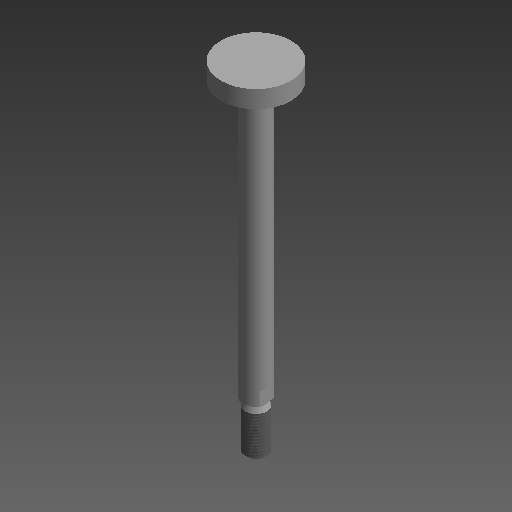
# Autodesk Inventor part: 193992 DSNU-32-60-PPS---(A---00--0-KS)
Saved by Autodesk Inventor 2021 (Build 250183000, 183)
## iProperties
Part Number: 193992 DSNU-32-60-PPS---(A---00--0-KS)
Material: Generic
Catalog Web Link: www.cadenas.de
Description: DSNU---(KS)-Standard cylinder
Vendor: FESTO
Document SubType Name: Modeling
Designer: partserver
Manufacturer: FESTO
Mass: 22.1775 g
Surface Area: 78.0411 cm^2
Volume: 22.1775 cm^3
Density: 1 g/cm^3
Appearance: PSOLRGB-192-192-192
Category: PARTsolutions
Company: FESTO
PSOL_IDENT_0: {$CADENAS_DATA\23d-libs\festo\parts\d\dsnu\parts\dsnu_metric_ks.prj},258 {VTYP=3D},{NB=193992 DSNU-3
PSOL_IDENT_1: 2-60-PPS---(A---00--0-KS)},{LINA=193992 DSNU-32-60-PPS},{NN=DSNU---(KS)},{DATE=25.01.2021 09:43:10},
PSOL_IDENT_2: {GEOMDATE=06.03.2020 09:03:14},{VERSION=},{LINEID=70},{WBVAR=TNR,HUB,DA,PE,ZD,VS,KA,K2A,K6,K3,K5,K8,
PSOL_IDENT_3: KP},{WBNUMERIC=HUB,K2A,K6,K8}  {NB=193992 DSNU-32-60-PPS---(A---00--0-KS)},{LINA=193992 DSNU-32-60-P
PSOL_IDENT_4: PS},{KT=DUMMY},{TNR=193992},{TYP=DSNU-32},{DSNU=METRIC},{KDM=32},{HUB=60},{DA=PPS},{DA1='P','PPV','P
PSOL_IDENT_5: PS'},{PE=A},{ZD=-},{VS=-},{VSALG='-','Q'},{KA=-},{KAALG='-','S2'},{K2A=0},{K6=0},{K3=-},{K31='-','K3'
PSOL_IDENT_6: },{K5=-},{K51='-','M10'},{K8=0},{KP=-},{KPALG='-','KP'},{A1=35},{A2=500},{A3=8},{A4=55.5},{AB=30},{A
PSOL_IDENT_7: M=22},{B=30},{BB=4},{BE=M30x1,5},{BENDM=30.000},{BEKDM=28.160},{BEP=1.500},{BS=6.6},{B1=48},{B2=10},
PSOL_IDENT_8: {B3=30},{B4=9},{B5=25.0},{B6=11},{B7=3},{CD=10},{D=38},{D1=30},{D2=12},{D3=33.6},{D4=10.0},{D5=34.0}
PSOL_IDENT_9: ,{D6=42},{D7=30},{EE=G1/8},{EENDM=9.728},{EEKDM=8.566},{EW=16},{F=38},{FF=M5},{FFNDM=5.000},{FFKDM=4
PSOL_IDENT_10: .019},{F1=19},{H=40},{H1=6},{KK=M10x1.25},{KKNDM=10.000},{KKKDM=0.000},{KKP=1.250},{K1=M6},{K1NDM=6.
PSOL_IDENT_11: 000},{K1KDM=4.773},{K2=2.5},{KV=0},{KW=8},{L=13},{LH=12.0},{LK=15.0},{L1=129.5},{L2=69.5},{L3=9.0},{
PSOL_IDENT_12: L4=26.0},{L5=24},{L6=56},{L7=30},{L8=19.0},{L9=25.0},{L10=85.5},{L11=97.5},{L12=65.5},{L13=137.5},{S
PSOL_IDENT_13: T=6.8},{SW=10},{T=12},{WH=34},{X=2.6},{XC=117.5},{K1KP=46},{K2KP=M5},{K2KPNDM=5.000},{K3KP=12},{K4KP=
PSOL_IDENT_14: 23.0},{K5KP=67.5},{K6KP=4.4},{K7KP=20},{K8KP=30.0},{K9KP=12.5},{K10KP=5.0},{K11KP=15},{K12KP=M5},{K1
PSOL_IDENT_15: 2KPNDM=5.000},{K13KP=55},{ZRSTART=45},{MHL=35.000},{ZRL=31.5},{C=17.200},{WHX=12.000},{LD1=27.800},{
PSOL_IDENT_16: LD2=27.700},{AD1=11.000},{AD2=8.000},{AD3=8.500},{AD4=7.000},{AD5=10.500},{MH1=11.000},{MH2=2.100},{
PSOL_IDENT_17: MH3=15.200},{KP1=25.000},{KP2=26.000},{KP3=20.000},{KP4=20.000},{KP5=36.000},{KPC=18.000},{KPF=3.000
PSOL_IDENT_18: },{KPG=17.500},{KPH=62.000},{KPJ=19.500},{KPK=17.000},{KPL=4.500},{KPR3=1.000},{KPR=19.000},{KPS=16.
PSOL_IDENT_19: 000},{MLD1=45.000},{MLD2=40.000},{MLD3=5.000},{MLL1=14.000},{KL1=65},{KKC=8.4},{KKD=1.5},{KKF=0.6},{
PSOL_IDENT_20: SWL=6.000},{K3L=6.400},{HUB1=60},{FDTXF31=4.000},{FDTB31=5.000}
NB: 193992 DSNU-32-60-PPS---(A---00--0-KS)
NN: DSNU---(KS)
NT: Standard cylinder
NBSYN: $TNR. $TYP.-$HUB1.-$DA.---($PE.$ZD.$VS.$KA.$K2A.$K6.$K3.$K5.$K8.$KP.KS)
LINA: 193992 DSNU-32-60-PPS
CATALOG: Festo
TNR: 193992
TYP: DSNU-32
DSNU: METRIC
KDM: 32
HUB: 60
DA: PPS
DA1: 'P','PPV','PPS'
PE: A
ZD: -
VS: -
KA: -
K2A: 0
K6: 0
K3: -
K31: '-','K3'
K5: -
K51: '-','M10'
K8: 0
KP: -
A1: 35
A2: 500
A3: 8
A4: 55.5
AB: 30
AM: 22
B: 30
BB: 4
BE: M30x1,5
BENDM: 30
BEKDM: 28.16
BEP: 1.5
BS: 6.6
B1: 48
B2: 10
B3: 30
B4: 9
B5: 25
B6: 11
B7: 3
CD: 10
D: 38
D1: 30
D2: 12
D3: 33.6
D4: 10
D5: 34
D6: 42
D7: 30
EE: G1/8
EENDM: 9.728
EEKDM: 8.566
EW: 16
F: 38
FF: M5
FFNDM: 5
FFKDM: 4.019
F1: 19
H: 40
H1: 6
KK: M10x1.25
KKNDM: 10
KKKDM: 0
KKP: 1.25
K1: M6
K1NDM: 6
K1KDM: 4.773
K2: 2.5
KV: 0
KW: 8
L: 13
LH: 12
LK: 15
L3: 9
L4: 26
L5: 24
L6: 56
L7: 30
L8: 19
L9: 25
L13: 137.5
ST: 6.8
SW: 10
T: 12
X: 2.6
K1KP: 46
K2KP: M5
K2KPNDM: 5
K3KP: 12
K4KP: 23
K5KP: 67.5
K6KP: 4.4
K7KP: 20
K8KP: 30
K9KP: 12.5
K10KP: 5
K11KP: 15
K12KP: M5
K12KPNDM: 5
K13KP: 55
MHL: 35
C: 17.2
WHX: 12
LD1: 27.8
LD2: 27.7
AD1: 11
AD2: 8
AD3: 8.5
AD4: 7
AD5: 10.5
MH1: 11
MH2: 2.1
MH3: 15.2
KP1: 25
KP2: 26
KP3: 20
KP4: 20
KP5: 36
KPC: 18
KPF: 3
KPG: 17.5
KPH: 62
KPJ: 19.5
KPK: 17
KPL: 4.5
KPR3: 1
KPR: 19
KPS: 16
MLD1: 45
MLD2: 40
MLD3: 5
MLL1: 14
SWL: 6
K3L: 6.4
FDTXF31: 4
FDTB31: 5
SUPPLIER: FESTO
ARTICLENO: 193992 DSNU-32-60-PPS---(A---00--0-KS)
BOMINFO: 193992 DSNU-32-60-PPS
CREATOR: CADENAS GmbH
Title: 193992 DSNU-32-60-PPS
Author: Cadenas PARTsolutions
Comments: Standard cylinder
Autodesk Inventor part; units mm, degrees
sketch "Sketch_2" plane through (0, 0, 0) normal (1, 0, 0) x (0, 1, 0)
  line L0 (0, -125) -> (0, 8)
  line L1 (0, 8) -> (6, 8)
  line L2 (6, 8) -> (6, -117)
  line L3 (6, -117) -> (16, -117)
  line L4 (16, -117) -> (16, -125)
  line L5 (16, -125) -> (0, -125)
  line L6 (0, -125) -> (0, 8)
  constraints: 14 end point
revolve "Revolution1" add sketch "Sketch_2" angle 360 about axis through (0, 0, -125) along (0, 0, -1)
sketch "Sketch_6" plane through (0, 0, 0) normal (1, 0, 0) x (0, 1, 0)
  line L0 (0, 7) -> (0, 30)
  line L1 (0, 30) -> (4.233, 30)
  line L2 (4.233, 30) -> (5, 29.233)
  line L3 (5, 29.233) -> (5, 11.698)
  line L4 (5, 11.698) -> (4.2362, 9.5994)
  arc A0 (4.2362, 9.5994) -> (4.2, 9.3942) centre (4.8, 9.3942) ccw
  line L5 (4.2, 9.3942) -> (4.2, 8.6)
  arc A1 (4.2, 8.6) -> (4.8, 8) centre (4.8, 8.6) ccw
  line L6 (4.8, 8) -> (5, 8)
  line L7 (5, 8) -> (5, 7)
  line L8 (5, 7) -> (0, 7)
  line L9 (0, 7) -> (0, 30)
  constraints: 20 end point, 4 point on circle, 2 centre point
revolve "Revolution2" add sketch "Sketch_6" angle 360 about axis through (0, 0, 7) along (0, 0, -1)
thread "Thread1" size "M10x1.25" class "6g" standard "ISO Metric profile" full length
sketch "Sketch_7" plane through (0, 0, 2) normal (0, 0, 1) x (1, 0, 0)
  line L0 (-10, 20) -> (-10, -10)
  line L1 (-10, -10) -> (-5, -10)
  line L2 (-5, -10) -> (-5, 10)
  line L3 (-5, 10) -> (5, 10)
  line L4 (5, 10) -> (5, -10)
  line L5 (5, -10) -> (10, -10)
  line L6 (10, -10) -> (10, 20)
  line L7 (10, 20) -> (-10, 20)
  constraints: 16 end point
extrude "Extrusion1" cut sketch "Sketch_7" along normal blind 7
ref_plane "FDT_KSAUFSATZ_XY" through (0, 0, 17) normal (0, 0, 1) x (-1, 0, 0)
ref_plane "FDT_KSAUFSATZ_YZ" through (0, 0, 17) normal (-1, 0, 0) x (0, -1, 0)
ref_plane "FDT_KSAUFSATZ_ZX" through (0, 0, 17) normal (0, -1, 0) x (0, 0, 1)
ref_plane "FDT_NUT_XY" through (0, 0, 17) normal (0, 0, 1) x (-1, 0, 0)
ref_plane "FDT_NUT_YZ" through (0, 0, 17) normal (-1, 0, 0) x (0, -1, 0)
ref_plane "FDT_NUT_ZX" through (0, 0, 17) normal (0, -1, 0) x (0, 0, 1)
ref_plane "KS_XY" through (0, 0, 0) normal (0, 0, -1) x (1, 0, 0)
ref_plane "KS_YZ" through (0, 0, 0) normal (1, 0, 0) x (0, -1, 0)
ref_plane "KS_ZX" through (0, 0, 0) normal (0, -1, 0) x (0, 0, -1)
ref_plane "NUT1_XY" through (0, 0, 22) normal (0, 0, 1) x (1, 0, 0)
ref_plane "NUT1_YZ" through (0, 0, 22) normal (1, 0, 0) x (0, 1, 0)
ref_plane "NUT1_ZX" through (0, 0, 22) normal (0, 1, 0) x (0, 0, 1)
body "Solid1"
